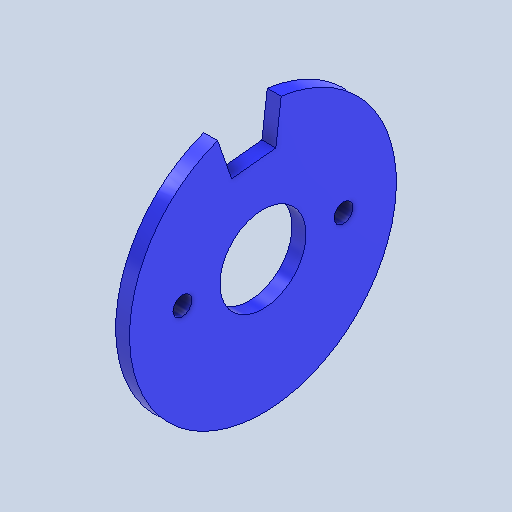
# Autodesk Inventor part: belt_liner_v2_3DP_P-3-F
Saved by Autodesk Inventor 2025.2 (Build 292293000, 293)
## iProperties
Created: 2025-01-13
Part Number: belt_liner_v2_3DP_P-3-F
Material: ABS プラスチック
Document SubType Name: Modeling
Designer: haruy
Density: 1.06 g/cm^3
Appearance: 青 - 壁塗料 - 光沢
Author: haruy
Autodesk Inventor part; units mm, degrees
ref_plane "YZ Plane" through (0, 0, 0) normal (1, 0, 0) x (0, 1, 0)
ref_plane "XZ Plane" through (0, 0, 0) normal (0, 1, 0) x (-1, 0, 0)
ref_plane "XY Plane" through (0, 0, 0) normal (0, 0, 1) x (1, 0, 0)
sketch "スケッチ1" plane through (0, 0, 0) normal (1, 0, 0) x (0, 1, 0)
  line L0 (18.91, 10.9564) -> (26.1282, 13.4771)
  arc A0 (26.1282, 13.4771) -> (27.3308, 2.0353) centre (3.5567, 5.3206) ccw
  line L1 (27.3308, 2.0353) -> (19.7463, 3.0002)
  line L2 (19.7463, 3.0002) -> (18.91, 10.9564)
  circle A1 centre (3.5567, 19.8206) radius 1.7
  circle A2 centre (3.5567, -9.1794) radius 1.7
  circle A3 centre (3.5567, 5.3206) radius 7.75
  point P0 (0, 0)
  constraints: 6 end point, 4 centre point, 2 point on circle
extrude "押し出し1" add sketch "スケッチ1" along normal blind 2.5
